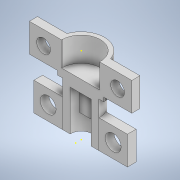
# Autodesk Inventor part: 4
Saved by Autodesk Inventor 2020.2 (Build 242310000, 310)
## iProperties
Created: 2020-02-07
Part Number: 4
Material: Generic
Document SubType Name: Modeling
Designer: ColinP
Density: 1 g/cm^3
Appearance: Default
Author: ColinP
Autodesk Inventor part; units mm, degrees
ref_plane "YZ Plane" through (0, 0, 0) normal (1, 0, 0) x (0, 1, 0)
ref_plane "XZ Plane" through (0, 0, 0) normal (0, 1, 0) x (-1, 0, 0)
ref_plane "XY Plane" through (0, 0, 0) normal (0, 0, 1) x (1, 0, 0)
sketch "Sketch3" plane through (0, 0, 0) normal (0, 1, 0) x (-1, 0, 0)
  circle A0 centre (0, 0) radius 4.5
  circle A1 centre (0, 0) radius 2.6
  dimension "d10" = 9
  dimension "d11" = 5.2
  constraints: 2 centre point, 2 coincident
  measures "d10" diameter of A0
  measures "d11" diameter of A1
extrude "Extrusion2" add sketch "Sketch3" along normal blind 4
sketch "Sketch4" plane through (0, 4, 0) normal (0, 1, 0) x (1, 0, 0)
  circle A0 centre (0, 0) radius 2.6 projected
  line L0 (0, -2.6) -> (0, -1.6)
  line L1 (0, -1.6) -> (0, 2.6)
  line L2 (0, -1.6) -> (-2.0494, -1.6)
  line L3 (0, -1.6) -> (2.0494, -1.6)
  line L4 (0, 2.6) -> (0, 2.6)
  line L5 (0, 2.6) -> (0, 2.6)
  circle A1 centre (0, 0) radius 4.5 projected
  circle A2 centre (0, 0) radius 2.6 projected
  line L6 (0, 2.6) -> (0, 1.6)
  line L7 (0, 1.6) -> (2.0494, 1.6)
  line L8 (0, 1.6) -> (-2.0494, 1.6)
  point P0 (2.0494, 1.6)
  point P1 (-2.0494, 1.6)
  dimension "d14" = 1
  dimension "d20" = 1
  constraints: 18 end point, 7 point on circle, 4 point on line, 1 horizontal, 1 midpoint, 1 parallel, 1 perpendicular, 1 vertical
  measures "d14" distance of L0.start L0.end
  measures "d20" distance of L5.end L6.end
extrude "Extrusion3" add sketch "Sketch4" along normal blind 6 contours L7 L1 A0 | A0 L0 L3 | L1 L8 A0 | A0 L2 L0 | A1
sketch "Sketch5" plane through (0, 10, 0) normal (0, 1, 0) x (1, 0, 0)
  circle A0 centre (0, 0) radius 4.5 projected
extrude "Extrusion4" add sketch "Sketch5" along normal blind 1
sketch "Sketch11" plane through (0, 0, 0) normal (0, -1, 0) x (1, 0, 0)
  point P0 (0, 0)
sketch "Sketch12" plane through (0, 11, 0) normal (0, 1, 0) x (1, 0, 0)
  circle A0 centre (0, 0) radius 4.685
  circle A1 centre (0, 0) radius 5.685
  dimension "d59" = 9.37
  dimension "d60" = 11.37
  constraints: 2 centre point, 2 coincident
  measures "d59" diameter of A0
  measures "d60" diameter of A1
extrude "Extrusion11" add sketch "Sketch12" along normal blind 2 contours A0 | A1
extrude "Extrusion12" add sketch "Sketch12" along normal blind 8
sketch "Sketch14" plane through (0, 19, 0) normal (0, 1, 0) x (1, 0, 0)
  point P0 (0, 0)
sketch "Sketch15" plane through (0, 19, 0) normal (0, 1, 0) x (1, 0, 0)
  circle A0 centre (0, 0) radius 5.685 projected
  line L0 (5.685, 0) -> (5.585, 0)
  line L1 (5.585, 0) -> (5.585, -1.0616)
  circle A1 centre (0, 0) radius 5.685 projected
  line L2 (5.585, 0) -> (5.585, 1.0616)
  line L3 (5.585, 1.0616) -> (12.585, 1.0616)
  line L4 (12.585, 1.0616) -> (12.585, -1.3379)
  line L5 (12.585, -1.3379) -> (5.585, -1.3379)
  line L6 (5.585, -1.3379) -> (5.585, 1.0616)
  line L7 (-5.6218, 0.8451) -> (-5.6218, -0.8451)
  line L8 (-5.6218, 0.8451) -> (-12.6218, 0.8451)
  line L9 (-12.6218, 0.8451) -> (-12.6218, -0.8451)
  line L10 (-12.6218, -0.8451) -> (-5.6218, -0.8451)
  line L11 (-5.6218, -0.8451) -> (-5.6218, 0.8451)
  point P0 (-5.6218, -0.8451)
  point P1 (8.9, -1.3379)
  point P2 (5.585, -1.0616)
  dimension "d72" = 0.1
  dimension "d73" = 7
  dimension "d74" = 7
  constraints: 24 end point, 5 point on circle, 4 parallel, 3 horizontal, 3 perpendicular, 2 vertical
  measures "d72" distance of L0.start L0.end
  measures "d73" distance of L4.end L5.end
  measures "d74" distance of L10.end L9.end
ref_plane "Work Plane3" through (-5.6218, 26, -0.8451) normal (0, 0, -1) x (-1, 0, 0)
sketch "Sketch17" plane through (-5.6218, 26, -0.8451) normal (0, 0, -1) x (-1, 0, 0)
  line L0 (7, 0) -> (7, -7) projected
  line L1 (-10.3068, 0) -> (7, 0) projected
  line L2 (7, -3.5) -> (3.5, -3.5)
  line L3 (-18.2068, 0) -> (-18.2068, -7) projected
  line L4 (-18.2068, -3.5) -> (-14.7068, -3.5)
  point P0 (-5.6218, -26)
  dimension "d81" = 3.5
  dimension "d82" = 3.5
  constraints: 4 end point, 2 horizontal, 2 midpoint
  measures "d81" distance of L2.start L2.end
  measures "d82" distance of L4.start L4.end
ref_plane "Work Plane2" through (7.7, 26, 0) normal (0, 0, 1) x (1, 0, 0)
sketch "Sketch19" plane through (7.7, 26, 0) normal (0, 0, 1) x (1, 0, 0)
  line L0 (-12.2, -26) -> (-12.2, -15) projected
  line L1 (-12.2, -26) -> (-19.2, -26)
  line L2 (-19.2, -26) -> (-19.2, -19)
  line L3 (-19.2, -19) -> (-12.2, -19)
  line L4 (-12.2, -19) -> (-12.2, -26)
  line L5 (-3.2, -15) -> (-3.2, -26) projected
  line L6 (-3.2, -26) -> (3.8, -26)
  line L7 (3.8, -26) -> (3.8, -19)
  line L8 (3.8, -19) -> (-3.2, -19)
  line L9 (-3.2, -19) -> (-3.2, -26)
  circle A0 centre (0.3, -22.5) radius 1.9558
  circle A1 centre (-15.7, -22.5) radius 1.9558
  point P0 (-7.7, -26)
  point P1 (-3.2, -19)
  dimension "d93" = 7
  dimension "d94" = 7
  dimension "d95" = 7
  dimension "d96" = 7
  dimension "d97" = 3.9116
  dimension "d98" = 3.9116
  constraints: 16 end point, 4 parallel, 2 centre point, 2 horizontal, 2 perpendicular
  measures "d93" distance of L2.end L3.end
  measures "d94" distance of L1.end L2.end
  measures "d95" distance of L8.end L7.end
  measures "d96" distance of L7.end L6.end
  measures "d97" diameter of A0
  measures "d98" diameter of A1
extrude "Extrusion17" add sketch "Sketch19" against normal blind 2
ref_plane "Work Plane1" through (7.7, 26, 0) normal (0, 0, 1) x (1, 0, 0)
sketch "Sketch20" plane through (7.7, 26, 0) normal (0, 0, 1) x (1, 0, 0)
  line L0 (-12.2, -19) -> (-12.2, -15) projected
  line L1 (-10.3, -16) -> (-10.3, -26) projected
  line L2 (-12.2, -19) -> (-10.3, -19)
  line L3 (-10.3, -19) -> (-10.3, -26)
  line L4 (-10.3, -26) -> (-12.2, -26)
  line L5 (-12.2, -26) -> (-12.2, -19)
  line L6 (-3.2, -26) -> (-5.1, -26) projected
  line L7 (-3.1953, -19) -> (-5.1, -19)
  line L8 (-5.1, -19) -> (-5.1, -26)
  line L9 (-5.1, -26) -> (-3.1953, -26)
  line L10 (-3.1953, -26) -> (-3.1953, -19)
  point P0 (-7.7, -26)
  constraints: 16 end point, 4 parallel, 2 horizontal, 2 perpendicular, 1 point on line
extrude "Extrusion18" add sketch "Sketch20" against normal blind 2
extrude "Extrusion20" add sketch "Sketch15" against normal blind 7 contours A0 L3 L4 L5 L6 | A0 L10 L9 L8
hole "Hole2" at (9.085, 22.5, -0.8451) at (-9.1218, 22.5, -0.8451) direction (0, 0, 1) diameter 3.4 end through all clearance for "Flat Head Machine Screw" size "M3" standard "Ansi Metric M Profile"
sketch "Sketch22" plane through (7.7, 26, 0) normal (0, 0, 1) x (1, 0, 0)
  point P0 (-7.7, -26)
sketch "Sketch23" plane through (5.585, 19, 1.3379) normal (0, 0, 1) x (1, 0, 0)
  point P0 (-5.585, -19)
sketch "Sketch24" plane through (12.585, 19, -1.0616) normal (0, 0, -1) x (-1, 0, 0)
  line L0 (0, 0) -> (0, -7) projected
  line L1 (0, 0) -> (7, 0) projected
  line L2 (0, -3.5) -> (3.5, -3.5)
  line L3 (3.5, -3.5) -> (3.5, 0)
  line L4 (3.5, 0) -> (0, 0)
  line L5 (0, 0) -> (0, -3.5)
  line L6 (18.2068, 0) -> (25.2068, 0) projected
  line L7 (25.2068, 0) -> (21.7068, 0)
  line L8 (21.7068, 0) -> (21.7068, -3.5)
  line L9 (21.7068, -3.5) -> (25.2068, -3.5)
  line L10 (25.2068, -3.5) -> (25.2068, 0)
  point P0 (12.585, -19)
  constraints: 16 end point, 4 parallel, 2 horizontal, 2 midpoint, 2 perpendicular
hole "Hole3" at (9.085, 15.5, -1.0616) at (-9.1218, 15.5, -1.0616) direction (0, 0, 1) diameter 3.4 end through all clearance for "Flat Head Machine Screw" size "M3" standard "Ansi Metric M Profile"
sketch "Sketch21" plane through (0, 19, 0) normal (0, 1, 0) x (1, 0, 0)
  line L0 (12.585, 1.0616) -> (12.585, -1.3379) projected
  line L1 (12.585, -0.1382) -> (-17.8482, -0.1382)
  line L2 (-17.8482, -0.1382) -> (-17.8482, -11.8989)
  line L3 (-17.8482, -11.8989) -> (12.585, -11.8989)
  line L4 (12.585, -11.8989) -> (12.585, -0.1382)
  point P0 (0, 0)
  constraints: 8 end point, 2 parallel, 1 horizontal, 1 midpoint, 1 perpendicular
extrude "Extrusion19" cut sketch "Sketch21" against normal blind 76.2
sketch "Sketch25" plane through (-12.6218, 19, 0.1382) normal (0, 0, 1) x (1, 0, 0)
  line L0 (7.9389, -6) -> (17.3048, -6) projected
  line L1 (17.3048, -6) -> (17.3048, -7)
  line L2 (25.2068, 0) -> (25.2068, -7) projected
  line L3 (17.3048, -7) -> (25.2068, -7)
  line L4 (25.2068, -7) -> (25.2068, 0)
  line L5 (25.2068, 0) -> (17.3048, 0)
  line L6 (17.3048, 0) -> (17.3048, -7)
  line L7 (7, 0) -> (0, 0) projected
  line L8 (7.9389, -7) -> (0, -7)
  line L9 (0, -7) -> (0, 0)
  line L10 (0, 0) -> (7.9389, 0)
  line L11 (7.9389, 0) -> (7.9389, -7)
  circle A0 centre (3.5, -3.5) radius 1.7 projected
  circle A1 centre (21.7068, -3.5) radius 1.7 projected
  point P0 (12.6218, -19)
  constraints: 18 end point, 4 parallel, 2 horizontal, 2 perpendicular, 1 point on line, 1 vertical
extrude "Extrusion21" add sketch "Sketch25" against normal blind 2
sketch "Sketch26" plane through (7.7, 26, 0) normal (0, 0, 1) x (1, 0, 0)
  line L0 (-19.2, -26) -> (-12.2, -26) projected
  line L1 (-12.2, -26) -> (-12.2, -19) projected
  line L2 (-12.2, -19) -> (-19.2, -19) projected
  line L3 (-19.2, -19) -> (-19.2, -26) projected
  circle A0 centre (-15.7, -22.5) radius 1.9558 projected
  circle A1 centre (0.3, -22.5) radius 1.9558 projected
  line L4 (-3.2, -26) -> (3.8, -26) projected
  line L5 (3.8, -26) -> (3.8, -19) projected
  line L6 (3.8, -19) -> (-3.2, -19) projected
  line L7 (-3.2, -26) -> (-3.2, -19) projected
  point P0 (-7.7, -26)
extrude "Extrusion22" add sketch "Sketch26" along normal up to surface (0.1382 mm away)
body "Solid2"
